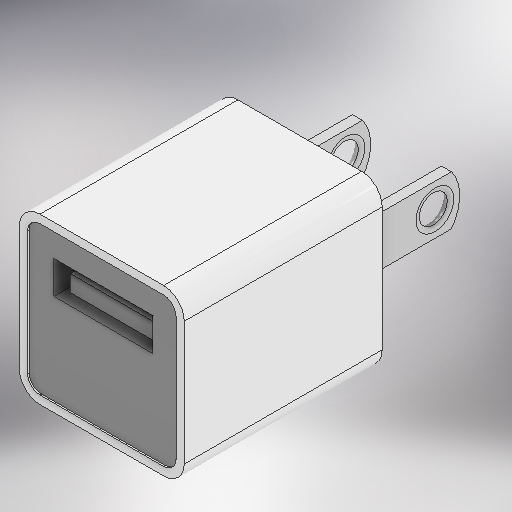
# Autodesk Inventor part: iPhone Charger
Saved by Autodesk Inventor 2026.2 (Build 302298000, 298)
## iProperties
Created: 2026-01-13
Part Number: iPhone Charger
Material: Generic
Document SubType Name: Modeling
Designer: andyeske
Density: 1 g/cm^3
Appearance: Default
Author: andyeske
Autodesk Inventor part; units mm, degrees
ref_plane "YZ Plane" through (0, 0, 0) normal (1, 0, 0) x (0, 1, 0)
ref_plane "XZ Plane" through (0, 0, 0) normal (0, 1, 0) x (-1, 0, 0)
ref_plane "XY Plane" through (0, 0, 0) normal (0, 0, 1) x (1, 0, 0)
sketch "Sketch1" plane through (0, 0, 0) normal (0, 0, 1) x (1, 0, 0)
  line L0 (-12.7, -12.7) -> (12.7, -12.7)
  line L1 (12.7, -12.7) -> (12.7, 12.7)
  line L2 (12.7, 12.7) -> (-12.7, 12.7)
  line L3 (-12.7, 12.7) -> (-12.7, -12.7)
  line L4 (-12.7, -12.7) -> (12.7, 12.7) construction
  line L5 (12.7, -12.7) -> (-12.7, 12.7) construction
  point P0 (0, 0)
  dimension "d0" = 25.4
  constraints: 12 end point, 2 midpoint, 2 parallel, 2 perpendicular, 1 horizontal
  measures "d0" distance of L2.end L0.start
extrude "Extrusion1" add sketch "Sketch1" along normal blind 30.48
fillet "Fillet1" radius 3.175 4 edges at (-12.7, 12.7, 15.24) (-12.7, -12.7, 15.24) (12.7, -12.7, 15.24) (12.7, 12.7, 15.24)
sketch "Sketch2" plane through (0, 0, 30.48) normal (0, 0, 1) x (1, 0, 0)
  arc A0 (12.7, 9.525) -> (9.525, 12.7) centre (9.525, 9.525) ccw projected
  line L0 (9.525, 12.7) -> (-9.525, 12.7) projected
  arc A1 (-9.525, 12.7) -> (-12.7, 9.525) centre (-9.525, 9.525) ccw projected
  line L1 (-12.7, 9.525) -> (-12.7, -9.525) projected
  arc A2 (-12.7, -9.525) -> (-9.525, -12.7) centre (-9.525, -9.525) ccw projected
  line L2 (-9.525, -12.7) -> (9.525, -12.7) projected
  arc A3 (9.525, -12.7) -> (12.7, -9.525) centre (9.525, -9.525) ccw projected
  line L3 (12.7, -9.525) -> (12.7, 9.525) projected
  line L4 (-9.525, 11.43) -> (9.525, 11.43)
  arc A4 (11.43, 9.525) -> (9.525, 11.43) centre (9.525, 9.525) ccw
  line L5 (11.43, 9.525) -> (11.43, -9.525)
  arc A5 (9.525, -11.43) -> (11.43, -9.525) centre (9.525, -9.525) ccw
  line L6 (9.525, -11.43) -> (-9.525, -11.43)
  arc A6 (-11.43, -9.525) -> (-9.525, -11.43) centre (-9.525, -9.525) ccw
  line L7 (-11.43, -9.525) -> (-11.43, 9.525)
  arc A7 (-9.525, 11.43) -> (-11.43, 9.525) centre (-9.525, 9.525) ccw
  point P0 (0, 0)
  dimension "d4" = 1.27
  constraints: 8 end point, 8 point on circle, 4 centre point, 7 other
  measures "d4" distance between parallel lines of L4 L0
extrude "Extrusion2" cut sketch "Sketch2" against normal blind 0.254 contours L4 A4 L5 A5 L6 A6 L7 A7
sketch "Sketch3" plane through (0, 0, 30.226) normal (0, 0, 1) x (1, 0, 0)
  line L0 (-7.62, 7.62) -> (7.62, 7.62)
  line L1 (7.62, 7.62) -> (7.62, 2.54)
  line L2 (7.62, 2.54) -> (-7.62, 2.54)
  line L3 (-7.62, 2.54) -> (-7.62, 7.62)
  line L4 (-7.62, 7.62) -> (7.62, 2.54) construction
  line L5 (7.62, 7.62) -> (-7.62, 2.54) construction
  line L6 (11.43, 9.525) -> (11.43, -9.525) projected
  line L7 (-11.43, -9.525) -> (-11.43, 9.525) projected
  line L8 (-9.525, 11.43) -> (9.525, 11.43) projected
  point P0 (0, 0)
  point P1 (0, 5.08)
  dimension "d7" = 3.81
  dimension "d8" = 3.81
  dimension "d9" = 3.81
  dimension "d10" = 5.08
  constraints: 12 end point, 2 midpoint, 2 parallel, 1 horizontal, 1 perpendicular
  measures "d7" distance between parallel lines of L6 L1
  measures "d8" distance between parallel lines of L7 L3
  measures "d9" distance between parallel lines of L8 L0
  measures "d10" distance of L2.end L0.start
extrude "Extrusion3" cut sketch "Sketch3" against normal blind 10.16
sketch "Sketch4" plane through (0, 0, 20.066) normal (0, 0, 1) x (1, 0, 0)
  line L0 (-6.35, 5.588) -> (6.35, 5.588)
  line L1 (6.35, 5.588) -> (6.35, 3.048)
  line L2 (6.35, 3.048) -> (-6.35, 3.048)
  line L3 (-6.35, 3.048) -> (-6.35, 5.588)
  line L4 (-6.35, 5.588) -> (6.35, 3.048) construction
  line L5 (6.35, 5.588) -> (-6.35, 3.048) construction
  line L6 (-7.62, 2.54) -> (-7.62, 7.62) projected
  line L7 (7.62, 7.62) -> (7.62, 2.54) projected
  line L8 (7.62, 2.54) -> (-7.62, 2.54) projected
  point P0 (0, 0)
  point P1 (0, 4.318)
  point P2 (7.62, 5.08)
  dimension "d13" = 1.27
  dimension "d14" = 1.27
  dimension "d15" = 0.508
  dimension "d16" = 2.54
  constraints: 12 end point, 3 midpoint, 2 parallel, 1 horizontal, 1 perpendicular
  measures "d13" distance between parallel lines of L6 L3
  measures "d14" distance from line of point (7.62, 5.08) L1
  measures "d15" distance between parallel lines of L8 L2
  measures "d16" distance of L0.end L1.end
extrude "Extrusion4" add sketch "Sketch4" along normal blind 8.89
sketch "Sketch5" plane through (0, 0, 0) normal (0, 0, -1) x (-1, 0, 0)
  line L0 (0, 0) -> (6.858, 0) construction
  line L1 (0, 0) -> (-6.858, 0) construction
  line L2 (6.096, -3.81) -> (7.62, -3.81)
  line L3 (7.62, -3.81) -> (7.62, 3.81)
  line L4 (7.62, 3.81) -> (6.096, 3.81)
  line L5 (6.096, 3.81) -> (6.096, -3.81)
  line L6 (6.096, -3.81) -> (7.62, 3.81) construction
  line L7 (7.62, -3.81) -> (6.096, 3.81) construction
  line L8 (-7.62, -3.81) -> (-6.096, -3.81)
  line L9 (-6.096, -3.81) -> (-6.096, 3.81)
  line L10 (-6.096, 3.81) -> (-7.62, 3.81)
  line L11 (-7.62, 3.81) -> (-7.62, -3.81)
  line L12 (-7.62, -3.81) -> (-6.096, 3.81) construction
  line L13 (-6.096, -3.81) -> (-7.62, 3.81) construction
  dimension "d19" = 6.858
  dimension "d20" = 7.62
  dimension "d21" = 1.524
  constraints: 28 end point, 4 horizontal, 4 midpoint, 4 parallel, 2 collinear, 2 perpendicular, 1 point on line
  measures "d19" distance of L0.start L0.end
  measures "d20" distance of L2.end L3.end
  measures "d21" distance of L3.end L4.end
extrude "Extrusion5" add sketch "Sketch5" along normal blind 17.78
sketch "Sketch6" plane through (-7.62, -3.81, 0) normal (-1, 0, 0) x (0, 0, 1)
  line L0 (0, 7.62) -> (-17.78, 7.62) projected
  line L1 (0, 0) -> (-17.78, 0) projected
  arc A0 (-15.748, 7.62) -> (-15.748, 0) centre (-10.668, 3.81) ccw
  line L2 (-15.748, 7.62) -> (-17.78, 7.62)
  line L3 (-17.78, 0) -> (-17.78, 7.62) projected
  line L4 (-17.78, 0) -> (-15.748, 0)
  point P0 (0, 3.81)
  dimension "d24" = 2.032
  dimension "d25" = 2.032
  dimension "d26" = 6.35
  constraints: 4 end point, 2 point on circle, 2 point on line, 1 centre point, 1 collinear, 1 perpendicular
  measures "d24" distance of L0.end L2.start
  measures "d25" distance of L1.end L4.end
  measures "d26" radius of A0
extrude "Extrusion6" cut sketch "Sketch6" against normal blind 17.78
sketch "Sketch7" plane through (-7.62, -3.81, 0) normal (-1, 0, 0) x (0, 0, 1)
  arc A0 (-15.748, 7.62) -> (-15.748, 0) centre (-10.668, 3.81) ccw construction
  line L0 (-17.018, 3.81) -> (-13.208, 3.81) construction
  circle A1 centre (-13.208, 3.81) radius 2.159
  point P0 (0, 3.81)
  dimension "d29" = 3.81
  dimension "d30" = 4.318
  constraints: 2 end point, 1 centre point, 1 coincident, 1 horizontal, 1 point on circle
  measures "d29" distance of L0.start L0.end
  measures "d30" diameter of A1
extrude "Extrusion7" cut sketch "Sketch7" against normal blind 17.78
fillet "Fillet2" radius 1.27 4 edges at (-7.62, 0, -15.367) (6.096, 0, -15.367) (-6.096, 0, -15.367) (7.62, 0, -15.367)
body "Solid1"
